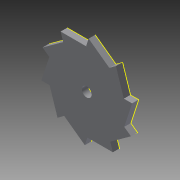
# Autodesk Inventor part: Part1
Saved by Autodesk Inventor 2013 (Build 170138000, 138)
## iProperties
Created: 2013-02-04
Part Number: Part1
Material: Generic
Document SubType Name: Modeling
Designer: Arpan
Density: 1 g/cm^3
Author: Arpan
Autodesk Inventor part; units mm, degrees
ref_plane "YZ Plane" through (0, 0, 0) normal (1, 0, 0) x (0, 1, 0)
ref_plane "XZ Plane" through (0, 0, 0) normal (0, 1, 0) x (-1, 0, 0)
ref_plane "XY Plane" through (0, 0, 0) normal (0, 0, 1) x (1, 0, 0)
sketch "Sketch1" plane through (0, 0, 0) normal (0, 0, 1) x (1, 0, 0)
  circle A0 centre (0, 0) radius 4.7625
  circle A1 centre (0, 0) radius 38.1
  line L0 (0, 38.1) -> (-25.4, 38.1)
  line L1 (0, 0) -> (-1.506, 4.5181)
  line L2 (-22.86, 30.48) -> (-25.4, 38.1)
  circle A2 centre (0, 0) radius 38.1
  line L3 (-22.3946, 30.8235) -> (-42.9436, 15.8938)
  line L4 (-36.4098, 11.2221) -> (-42.9436, 15.8938)
  circle A3 centre (0, 0) radius 38.1
  line L5 (-36.2353, 11.7735) -> (-44.0843, -12.3833)
  line L6 (-36.0523, -12.3223) -> (-44.0843, -12.3833)
  circle A4 centre (0, 0) radius 38.1
  line L7 (-36.2353, -11.7735) -> (-28.3862, -35.9304)
  line L8 (-21.9241, -31.16) -> (-28.3862, -35.9304)
  circle A5 centre (0, 0) radius 38.1
  line L9 (-22.3946, -30.8235) -> (-1.8456, -45.7533)
  line L10 (0.5784, -38.0956) -> (-1.8456, -45.7533)
  circle A6 centre (0, 0) radius 38.1
  line L11 (0, -38.1) -> (25.4, -38.1)
  line L12 (22.86, -30.48) -> (25.4, -38.1)
  circle A7 centre (0, 0) radius 38.1
  line L13 (22.3946, -30.8235) -> (42.9436, -15.8938)
  line L14 (36.4098, -11.2221) -> (42.9436, -15.8938)
  circle A8 centre (0, 0) radius 38.1
  line L15 (36.2353, -11.7735) -> (44.0843, 12.3833)
  line L16 (36.0523, 12.3223) -> (44.0843, 12.3833)
  circle A9 centre (0, 0) radius 38.1
  line L17 (36.2353, 11.7735) -> (28.3862, 35.9304)
  line L18 (21.9241, 31.16) -> (28.3862, 35.9304)
  circle A10 centre (0, 0) radius 38.1
  line L19 (22.3946, 30.8235) -> (1.8456, 45.7533)
  line L20 (-0.5784, 38.0956) -> (1.8456, 45.7533)
  dimension "d0" = 9.525
  dimension "d1" = 76.2
  dimension "d2" = 25.4
  dimension "d5" = 360
  constraints: 42 end point, 20 point on circle, 10 centre point, 2 coincident, 1 horizontal, 1 tangent, 74 other
  measures "d1" diameter of A1
  measures "d2" distance of L0.start L0.end
extrude "Extrusion1" add sketch "Sketch1" along normal blind 6.35
sketch "Sketch2" plane through (0, 0, 0) normal (0, 0, -1) x (-1, 0, 0)
  line L0 (-28.3862, 35.9304) -> (-21.9278, 31.1627) projected
  line L1 (-36.0569, 12.3223) -> (-28.3862, 35.9304) projected
  line L2 (-44.0843, 12.3833) -> (-36.0569, 12.3223) projected
  line L3 (-36.4136, -11.2247) -> (-44.0843, 12.3833) projected
  line L4 (-42.9436, -15.8938) -> (-36.4136, -11.2247) projected
  line L5 (-22.8615, -30.4844) -> (-42.9436, -15.8938) projected
  line L6 (-25.4, -38.1) -> (-22.8615, -30.4844) projected
  line L7 (-0.577, -38.1) -> (-25.4, -38.1) projected
  line L8 (1.8456, -45.7533) -> (-0.577, -38.1) projected
  line L9 (21.9278, -31.1627) -> (1.8456, -45.7533) projected
  line L10 (28.3862, -35.9304) -> (21.9278, -31.1627) projected
  line L11 (36.0569, -12.3223) -> (28.3862, -35.9304) projected
  line L12 (44.0843, -12.3833) -> (36.0569, -12.3223) projected
  line L13 (36.4136, 11.2247) -> (44.0843, -12.3833) projected
  line L14 (42.9436, 15.8938) -> (36.4136, 11.2247) projected
  line L15 (22.8615, 30.4844) -> (42.9436, 15.8938) projected
  line L16 (25.4, 38.1) -> (22.8615, 30.4844) projected
  line L17 (0.577, 38.1) -> (25.4, 38.1) projected
  line L18 (-1.8456, 45.7533) -> (0.577, 38.1) projected
  line L19 (-21.9278, 31.1627) -> (-1.8456, 45.7533) projected
  circle A0 centre (0, 0) radius 4.7625 projected
body "Solid1"
